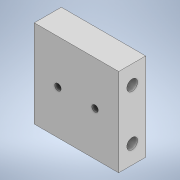
# Autodesk Inventor part: Soporte barras
Saved by Autodesk Inventor 2021 (Build 250183000, 183)
## iProperties
Created: 2021-05-29
Part Number: Soporte barras
Material: Generic
Document SubType Name: Modeling
Designer: Nelson
Density: 1 g/cm^3
Appearance: Default
Author: Nelson
Autodesk Inventor part; units mm, degrees
ref_plane "YZ Plane" through (0, 0, 0) normal (1, 0, 0) x (0, 1, 0)
ref_plane "XZ Plane" through (0, 0, 0) normal (0, 1, 0) x (-1, 0, 0)
ref_plane "XY Plane" through (0, 0, 0) normal (0, 0, 1) x (1, 0, 0)
sketch "Sketch1" plane through (0, 0, 0) normal (0, 0, 1) x (1, 0, 0)
  line L0 (0, 0) -> (250, 0)
  line L1 (250, 0) -> (250, 260)
  line L2 (250, 260) -> (0, 260)
  line L3 (0, 260) -> (0, 0)
  dimension "d0" = 250
  dimension "d1" = 260
  constraints: 8 end point, 2 parallel, 1 horizontal, 1 perpendicular
  measures "d0" distance of L1.end L2.end
  measures "d1" distance of L0.end L1.end
extrude "Extrusion1" add sketch "Sketch1" against normal blind 80
sketch "Sketch2" plane through (250, 0, 0) normal (1, 0, 0) x (0, 0, -1)
  line L0 (0, 0) -> (0, 260) projected
  line L1 (0, 260) -> (80, 260) projected
  point P0 (40, 205)
  point P1 (40, 55)
  dimension "d4" = 40
  dimension "d5" = 40
  dimension "d6" = 150
  dimension "d7" = 55
  measures "d4" distance from line of point (40, 205) L0
  measures "d5" distance from line of point (40, 55) L0
  measures "d6" distance of point (40, 55) point (40, 205)
  measures "d7" distance from line of L1 point (40, 205)
hole "Hole1" at (250, 205, -40) at (250, 55, -40) direction (-1, 0, 0) diameter 32 end through all
sketch "Sketch3" plane through (0, 0, 0) normal (0, 0, 1) x (1, 0, 0)
  line L0 (0, 0) -> (250, 0) projected
  line L1 (250, 260) -> (0, 260) projected
  line L2 (0, 260) -> (0, 0) projected
  line L3 (250, 0) -> (250, 260) projected
  point P0 (70, 130)
  point P1 (180, 130)
  dimension "d16" = 130
  dimension "d17" = 130
  dimension "d18" = 70
  dimension "d19" = 70
  measures "d16" distance from line of point (70, 130) L1
  measures "d17" distance from line of L1 point (180, 130)
  measures "d18" distance from line of point (70, 130) L2
  measures "d19" distance from line of L3 point (180, 130)
hole "Hole2" at (70, 130, 0) at (180, 130, 0) direction (0, 0, -1) diameter 19.177 end through all thread size "7/8-9 UNC" class "2B" standard "ANSI Unified Screw Threads"
equation "\"d5\" = d4"
equation "\"d17\" = d16"
equation "\"d19\" = d18"
body "Solid1"
